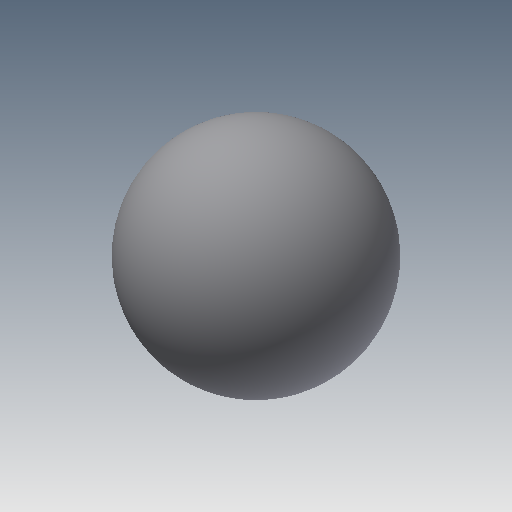
# Autodesk Inventor part: 676A Ball
Saved by Autodesk Inventor 2019.4 (Build 234330000, 330)
## iProperties
Category: PARTsolutions
Company: NTN
Created: 2019-06-11
Part Number: 676A Ball
Material: 一般
Catalog Web Link: www.cadenas.de
Description: Six types ball-Metric system sizes
Vendor: NTN
Document SubType Name: Modeling
Designer: psadmin
Manufacturer: NTN
Mass: 0.000869068 g
Surface Area: 0.0440406 cm^2
Volume: 0.000869068 cm^3
Density: 1 g/cm^3
Appearance: PSOLRGB-192-192-192
PSOL_IDENT_0: {$CADENAS_DATA\23d-libs\ntn\ball_roller_bearings\miniature_extra_small_bb\metric_system_sizes\mss_ba
PSOL_IDENT_1: ll.prj},168 {VTYP=3D},{NB=676A Ball},{LINA=676A Ball},{NN=Six types ball},{DATE=29.01.2019 23:03:32}
PSOL_IDENT_2: ,{GEOMDATE=02.04.2007 00:00:00},{VERSION=},{LINEID=9710},{WBVAR=},{WBNUMERIC=}  {NB=676A Ball},{LINA=
PSOL_IDENT_3: 676A Ball},{KT=DUMMY},{IDNR=},{SD=6.0},{D=10},{B=2.5},{R=0.10},{ORDER=676A},{CR=465},{COR=196},{CRF=
PSOL_IDENT_4: 47},{CORF=20},{LSG=43 000},{LSO=51 000},{MASS=0.65},{ORDER1=676A},{D1=11.2},{D2=11.2},{C1=0.6},{C2=0
PSOL_IDENT_5: .6},{WSS=WA676AZ},{WDS=ZZ},{UTWF=FL676A},{FORSS=FLWA676AZ},{FORDS=ZZ},{DA1=6,6},{DA2=6,7},{DA=9,2},{
PSOL_IDENT_6: RAS=0,1},{MASS1=0.74},{B1=3.0},{VERS=1},{X=2},{N=12},{O=25.12},{RB=0.592}
NN: Six types ball
NT: Metric system sizes
NB: 676A Ball
NBSYN: $ORDER. Ball
LINA: 676A Ball
SD: 6
D: 10
B: 2.5
R: 0.1
CR: 465
COR: 196
CRF: 47
CORF: 20
LSG: 43 000
LSO: 51 000
MASS: 0.65
ORDER1: 676A
D1: 11.2
D2: 11.2
C1: 0.6
C2: 0.6
WSS: WA676AZ
WDS: ZZ
UTWF: FL676A
FORSS: FLWA676AZ
FORDS: ZZ
DA1: 6,6
DA2: 6,7
DA: 9,2
RAS: 0,1
MASS1: 0.74
B1: 3
VERS: 1
SUPPLIER: NTN
ARTICLENO: 676A Ball
BOMINFO: 676A Ball
CREATOR: CADENAS GmbH
Title: 676A Ball
Author: Cadenas PARTsolutions
Comments: Metric system sizes
Autodesk Inventor part; units mm, degrees
sketch "Sketch_1" plane through (0, 0, 0) normal (0, 0, 1) x (1, 0, 0)
  line L0 (0.592, 0) -> (-0.592, 0)
  arc A0 (0.592, 0) -> (-0.592, 0) centre (0, 0) ccw
  line L1 (0.592, 0) -> (-0.592, 0)
  constraints: 4 end point, 2 point on circle, 1 centre point
revolve "Revolution1" add sketch "Sketch_1" angle 360 about axis through (0.592, 0, 0) along (1, 0, 0)
ref_plane "mss_ball_XY" through (0, 0, 0) normal (1, 0, 0) x (0, 0, -1)
ref_plane "mss_ball_YZ" through (0, 0, 0) normal (0, 0, -1) x (0, 1, 0)
ref_plane "mss_ball_ZX" through (0, 0, 0) normal (0, 1, 0) x (1, 0, 0)
body "Solid1"
